Autodesk Inventor part; units mm, degrees
(part 2 of 5)
  spline S151 degree 2 poles (-398.6924, 73.057) (-398.9442, 73.057) (-399.3064, 73.4191) (-399.3064, 73.6794) knots 0 0 0 1 2 2 2
  spline S152 degree 2 poles (-399.3064, 73.6794) (-399.3064, 73.9312) (-398.9499, 74.2934) (-398.6924, 74.2934) knots 0 0 0 1 2 2 2
  spline S153 degree 2 poles (-398.6924, 74.2934) (-398.4293, 74.2934) (-398.07, 73.9256) (-398.07, 73.6794) knots 0 0 0 1 2 2 2
  line L183 (-388.2805, 72.641) -> (-388.4135, 73.2013)
  line L184 (-388.4135, 73.2013) -> (-389.3246, 73.2013)
  line L185 (-389.3246, 73.2013) -> (-389.4689, 72.641)
  line L186 (-389.4689, 72.641) -> (-390.4619, 72.641)
  line L187 (-390.4619, 72.641) -> (-389.4123, 75.691)
  line L188 (-389.4123, 75.691) -> (-388.2721, 75.691)
  line L189 (-388.2721, 75.691) -> (-387.2818, 72.641)
  line L190 (-387.2818, 72.641) -> (-388.2805, 72.641)
  line L191 (-388.8577, 75.0262) -> (-388.8775, 75.0262)
  spline S154 degree 2 poles (-388.8775, 75.0262) (-388.8832, 74.9752) (-388.9341, 74.7404) (-389.1661, 73.8548) knots 0 0 0 1 2 2 2
  line L192 (-389.1661, 73.8548) -> (-388.5833, 73.8548)
  line L193 (-388.5833, 73.8548) -> (-388.7955, 74.6838)
  spline S155 degree 2 poles (-388.7955, 74.6838) (-388.8407, 74.8677) (-388.8577, 75.0262) knots 0 0 0 1 1 1
  line L194 (-385.5955, 72.641) -> (-385.5955, 73.8294)
  spline S156 degree 2 poles (-385.5955, 73.8294) (-385.5955, 74.0331) (-385.7172, 74.2085) (-385.853, 74.2085) knots 0 0 0 1 2 2 2
  spline S157 degree 2 poles (-385.853, 74.2085) (-385.969, 74.2085) (-386.102, 74.0246) (-386.102, 73.8831) knots 0 0 0 1 2 2 2
  line L195 (-386.102, 73.8831) -> (-386.102, 72.641)
  line L196 (-386.102, 72.641) -> (-387.0074, 72.641)
  line L197 (-387.0074, 72.641) -> (-387.0074, 74.8196)
  line L198 (-387.0074, 74.8196) -> (-386.102, 74.8196)
  line L199 (-386.102, 74.8196) -> (-386.102, 74.4801)
  line L200 (-386.102, 74.4801) -> (-386.0935, 74.4801)
  spline S158 degree 2 poles (-386.0935, 74.4801) (-385.986, 74.6668) (-385.6182, 74.8734) (-385.4031, 74.8734) knots 0 0 0 1 2 2 2
  spline S159 degree 2 poles (-385.4031, 74.8734) (-384.6901, 74.8734) (-384.6901, 73.9708) knots 0 0 0 1 1 1
  line L201 (-384.6901, 73.9708) -> (-384.6901, 72.641)
  line L202 (-384.6901, 72.641) -> (-385.5955, 72.641)
  spline S160 degree 2 poles (-381.9174, 72.9438) (-381.9174, 72.3157) (-382.7068, 71.6168) (-383.465, 71.6168) knots 0 0 0 1 2 2 2
  spline S161 degree 2 poles (-383.465, 71.6168) (-383.6688, 71.6168) (-384.0535, 71.6819) (-384.1356, 71.7215) knots 0 0 0 1 2 2 2
  line L203 (-384.1356, 71.7215) -> (-384.1356, 72.4317)
  spline S162 degree 2 poles (-384.1356, 72.4317) (-383.9998, 72.3468) (-383.632, 72.2449) (-383.4905, 72.2449) knots 0 0 0 1 2 2 2
  spline S163 degree 2 poles (-383.4905, 72.2449) (-383.1849, 72.2449) (-382.82, 72.5392) (-382.82, 72.7825) knots 0 0 0 1 2 2 2
  line L204 (-382.82, 72.7825) -> (-382.82, 72.9155)
  line L205 (-382.82, 72.9155) -> (-382.8285, 72.9155)
  spline S164 degree 2 poles (-382.8285, 72.9155) (-382.9275, 72.7655) (-383.2698, 72.5873) (-383.465, 72.5873) knots 0 0 0 1 2 2 2
  spline S165 degree 2 poles (-383.465, 72.5873) (-383.8866, 72.5873) (-384.3761, 73.173) (-384.3761, 73.6879) knots 0 0 0 1 2 2 2
  spline S166 degree 2 poles (-384.3761, 73.6879) (-384.3761, 74.0416) (-384.1215, 74.582) (-383.6659, 74.8734) (-383.3915, 74.8734) knots 0 0 0 1 2 3 3 3
  spline S167 degree 2 poles (-383.3915, 74.8734) (-383.0124, 74.8734) (-382.8285, 74.5933) knots 0 0 0 1 1 1
  line L206 (-382.8285, 74.5933) -> (-382.82, 74.5933)
  line L207 (-382.82, 74.5933) -> (-382.82, 74.8196)
  line L208 (-382.82, 74.8196) -> (-381.9174, 74.8196)
  line L209 (-381.9174, 74.8196) -> (-381.9174, 72.9438)
  spline S168 degree 2 poles (-382.8058, 73.7926) (-382.8058, 73.9821) (-382.9784, 74.2085) (-383.1199, 74.2085) knots 0 0 0 1 2 2 2
  spline S169 degree 2 poles (-383.1199, 74.2085) (-383.2727, 74.2085) (-383.4566, 73.9369) (-383.4566, 73.7077) knots 0 0 0 1 2 2 2
  spline S170 degree 2 poles (-383.4566, 73.7077) (-383.4566, 73.4983) (-383.3038, 73.2522) (-383.1368, 73.2522) knots 0 0 0 1 2 2 2
  spline S171 degree 2 poles (-383.1368, 73.2522) (-382.9812, 73.2522) (-382.8058, 73.504) (-382.8058, 73.719) knots 0 0 0 1 2 2 2
  line L210 (-382.8058, 73.719) -> (-382.8058, 73.7926)
  spline S172 degree 2 poles (-380.7008, 73.4729) (-380.6782, 73.3314) (-380.4009, 73.173) (-380.1746, 73.173) knots 0 0 0 1 2 2 2
  spline S173 degree 2 poles (-380.1746, 73.173) (-379.8577, 73.173) (-379.5747, 73.2946) knots 0 0 0 1 1 1
  line L211 (-379.5747, 73.2946) -> (-379.5747, 72.7203)
  spline S174 degree 2 poles (-379.5747, 72.7203) (-379.9029, 72.5873) (-380.3754, 72.5873) knots 0 0 0 1 1 1
  spline S175 degree 2 poles (-380.3754, 72.5873) (-380.9441, 72.5873) (-381.5779, 73.1701) (-381.5779, 73.6822) knots 0 0 0 1 2 2 2
  spline S176 degree 2 poles (-381.5779, 73.6822) (-381.5779, 74.0331) (-381.3006, 74.5678) (-380.7546, 74.8734) (-380.4235, 74.8734) knots 0 0 0 1 2 3 3 3
  spline S177 degree 2 poles (-380.4235, 74.8734) (-380.0868, 74.8734) (-379.6059, 74.6103) (-379.3569, 74.1321) (-379.3569, 73.8124) knots 0 0 0 1 2 3 3 3
  line L212 (-379.3569, 73.8124) -> (-379.3569, 73.4729)
  line L213 (-379.3569, 73.4729) -> (-380.7008, 73.4729)
  spline S178 degree 2 poles (-380.1576, 73.9482) (-380.1576, 74.3245) (-380.4264, 74.3245) knots 0 0 0 1 1 1
  spline S179 degree 2 poles (-380.4264, 74.3245) (-380.5395, 74.3245) (-380.6923, 74.118) (-380.7065, 73.9482) knots 0 0 0 1 2 2 2
  line L214 (-380.7065, 73.9482) -> (-380.1576, 73.9482)
  line L215 (-379.0428, 72.641) -> (-379.0428, 75.8665)
  line L216 (-379.0428, 75.8665) -> (-378.1375, 75.8665)
  line L217 (-378.1375, 75.8665) -> (-378.1375, 72.641)
  line L218 (-378.1375, 72.641) -> (-379.0428, 72.641)
  spline S180 degree 2 poles (-375.2798, 73.7699) (-375.2798, 73.2182) (-375.9447, 72.5873) (-376.5417, 72.5873) knots 0 0 0 1 2 2 2
  spline S181 degree 2 poles (-376.5417, 72.5873) (-377.1359, 72.5873) (-377.7979, 73.2013) (-377.7979, 73.7445) knots 0 0 0 1 2 2 2
  spline S182 degree 2 poles (-377.7979, 73.7445) (-377.7979, 74.0897) (-377.4867, 74.6018) (-376.9124, 74.8734) (-376.5389, 74.8734) knots 0 0 0 1 2 3 3 3
  spline S183 degree 2 poles (-376.5389, 74.8734) (-376.1513, 74.8734) (-375.5826, 74.5876) (-375.2798, 74.0812) (-375.2798, 73.7699) knots 0 0 0 1 2 3 3 3
  spline S184 degree 2 poles (-376.1994, 73.7643) (-376.1994, 74.2085) (-376.5389, 74.2085) knots 0 0 0 1 1 1
  spline S185 degree 2 poles (-376.5389, 74.2085) (-376.8784, 74.2085) (-376.8784, 73.7445) knots 0 0 0 1 1 1
  spline S186 degree 2 poles (-376.8784, 73.7445) (-376.8784, 73.2522) (-376.5332, 73.2522) knots 0 0 0 1 1 1
  spline S187 degree 2 poles (-376.5332, 73.2522) (-376.1994, 73.2522) (-376.1994, 73.7643) knots 0 0 0 1 1 1
  line L219 (-373.5285, 72.641) -> (-373.5285, 73.8294)
  spline S188 degree 2 poles (-373.5285, 73.8294) (-373.5285, 74.0331) (-373.6502, 74.2085) (-373.786, 74.2085) knots 0 0 0 1 2 2 2
  spline S189 degree 2 poles (-373.786, 74.2085) (-373.902, 74.2085) (-374.0349, 74.0246) (-374.0349, 73.8831) knots 0 0 0 1 2 2 2
  line L220 (-374.0349, 73.8831) -> (-374.0349, 72.641)
  line L221 (-374.0349, 72.641) -> (-374.9403, 72.641)
  line L222 (-374.9403, 72.641) -> (-374.9403, 74.8196)
  line L223 (-374.9403, 74.8196) -> (-374.0349, 74.8196)
  line L224 (-374.0349, 74.8196) -> (-374.0349, 74.4801)
  line L225 (-374.0349, 74.4801) -> (-374.0265, 74.4801)
  spline S190 degree 2 poles (-374.0265, 74.4801) (-373.9189, 74.6668) (-373.5511, 74.8734) (-373.3361, 74.8734) knots 0 0 0 1 2 2 2
  spline S191 degree 2 poles (-373.3361, 74.8734) (-372.6231, 74.8734) (-372.6231, 73.9708) knots 0 0 0 1 1 1
  line L226 (-372.6231, 73.9708) -> (-372.6231, 72.641)
  line L227 (-372.6231, 72.641) -> (-373.5285, 72.641)
  line L228 (-372.2129, 72.641) -> (-372.2129, 74.8196)
  line L229 (-372.2129, 74.8196) -> (-371.3075, 74.8196)
  line L230 (-371.3075, 74.8196) -> (-371.3075, 72.641)
  line L231 (-371.3075, 72.641) -> (-372.2129, 72.641)
  spline S192 degree 2 poles (-371.2537, 75.4081) (-371.2537, 75.2157) (-371.5338, 74.9781) (-371.7602, 74.9781) knots 0 0 0 1 2 2 2
  spline S193 degree 2 poles (-371.7602, 74.9781) (-371.9809, 74.9781) (-372.2638, 75.2242) (-372.2638, 75.4081) knots 0 0 0 1 2 2 2
  spline S194 degree 2 poles (-372.2638, 75.4081) (-372.2638, 75.5949) (-371.9894, 75.8269) (-371.7602, 75.8269) knots 0 0 0 1 2 2 2
  spline S195 degree 2 poles (-371.7602, 75.8269) (-371.5338, 75.8269) (-371.2537, 75.5949) (-371.2537, 75.4081) knots 0 0 0 1 2 2 2
  line L232 (-369.5788, 72.641) -> (-369.5788, 75.691)
  line L233 (-369.5788, 75.691) -> (-368.6593, 75.691)
  line L234 (-368.6593, 75.691) -> (-368.6593, 72.641)
  line L235 (-368.6593, 72.641) -> (-369.5788, 72.641)
  line L236 (-368.1415, 72.641) -> (-368.1415, 75.8665)
  line L237 (-368.1415, 75.8665) -> (-367.2361, 75.8665)
  line L238 (-367.2361, 75.8665) -> (-367.2361, 72.641)
  line L239 (-367.2361, 72.641) -> (-368.1415, 72.641)
  line L240 (-365.5923, 72.641) -> (-365.5923, 72.9721)
  line L241 (-365.5923, 72.9721) -> (-365.6008, 72.9721)
  spline S196 degree 2 poles (-365.6008, 72.9721) (-365.8186, 72.5873) (-366.2657, 72.5873) knots 0 0 0 1 1 1
  spline S197 degree 2 poles (-366.2657, 72.5873) (-366.574, 72.5873) (-366.9221, 72.9523) (-366.9221, 73.2607) knots 0 0 0 1 2 2 2
  spline S198 degree 2 poles (-366.9221, 73.2607) (-366.9221, 73.9029) (-366.1327, 74.0048) knots 0 0 0 1 1 1
  line L242 (-366.1327, 74.0048) -> (-365.5923, 74.0755)
  spline S199 degree 2 poles (-365.5923, 74.0755) (-365.5923, 74.183) (-365.7847, 74.3188) (-365.9459, 74.3188) knots 0 0 0 1 2 2 2
  spline S200 degree 2 poles (-365.9459, 74.3188) (-366.3109, 74.3188) (-366.7183, 74.1095) knots 0 0 0 1 1 1
  line L243 (-366.7183, 74.1095) -> (-366.7183, 74.698)
  spline S201 degree 2 poles (-366.7183, 74.698) (-366.5429, 74.7744) (-366.0082, 74.8734) (-365.8186, 74.8734) knots 0 0 0 1 2 2 2
  spline S202 degree 2 poles (-365.8186, 74.8734) (-365.2641, 74.8734) (-364.7633, 74.3981) (-364.7633, 73.8435) knots 0 0 0 1 2 2 2
  line L244 (-364.7633, 73.8435) -> (-364.7633, 72.641)
  line L245 (-364.7633, 72.641) -> (-365.5923, 72.641)
  spline S203 degree 2 poles (-366.1298, 73.3823) (-366.1298, 73.2946) (-366.0167, 73.1786) (-365.912, 73.1786) knots 0 0 0 1 2 2 2
  spline S204 degree 2 poles (-365.912, 73.1786) (-365.7705, 73.1786) (-365.5923, 73.3908) (-365.5923, 73.5577) knots 0 0 0 1 2 2 2
  line L246 (-365.5923, 73.5577) -> (-365.5923, 73.6398)
  line L247 (-365.5923, 73.6398) -> (-365.9007, 73.5974)
  spline S205 degree 2 poles (-365.9007, 73.5974) (-366.1298, 73.5577) (-366.1298, 73.3823) knots 0 0 0 1 1 1
  spline S206 degree 2 poles (-362.7177, 74.0444) (-362.7686, 74.067) (-362.944, 74.1038) (-363.0006, 74.1038) knots 0 0 0 1 2 2 2
  spline S207 degree 2 poles (-363.0006, 74.1038) (-363.4505, 74.1038) (-363.4505, 73.586) knots 0 0 0 1 1 1
  line L248 (-363.4505, 73.586) -> (-363.4505, 72.641)
  line L249 (-363.4505, 72.641) -> (-364.3559, 72.641)
  line L250 (-364.3559, 72.641) -> (-364.3559, 74.8196)
  line L251 (-364.3559, 74.8196) -> (-363.4505, 74.8196)
  line L252 (-363.4505, 74.8196) -> (-363.4505, 74.4377)
  line L253 (-363.4505, 74.4377) -> (-363.442, 74.4377)
  spline S208 degree 2 poles (-363.442, 74.4377) (-363.3599, 74.6442) (-363.0516, 74.8592) (-362.8478, 74.8592) knots 0 0 0 1 2 2 2
  spline S209 degree 2 poles (-362.8478, 74.8592) (-362.7743, 74.8592) (-362.7177, 74.8338) knots 0 0 0 1 1 1
  line L254 (-362.7177, 74.8338) -> (-362.7177, 74.0444)
  line L255 (-362.4574, 72.641) -> (-362.4574, 74.8196)
  line L256 (-362.4574, 74.8196) -> (-361.552, 74.8196)
  line L257 (-361.552, 74.8196) -> (-361.552, 72.641)
  line L258 (-361.552, 72.641) -> (-362.4574, 72.641)
  spline S210 degree 2 poles (-361.4983, 75.4081) (-361.4983, 75.2157) (-361.7784, 74.9781) (-362.0047, 74.9781) knots 0 0 0 1 2 2 2
  spline S211 degree 2 poles (-362.0047, 74.9781) (-362.2254, 74.9781) (-362.5083, 75.2242) (-362.5083, 75.4081) knots 0 0 0 1 2 2 2
  spline S212 degree 2 poles (-362.5083, 75.4081) (-362.5083, 75.5949) (-362.2339, 75.8269) (-362.0047, 75.8269) knots 0 0 0 1 2 2 2
  spline S213 degree 2 poles (-362.0047, 75.8269) (-361.7784, 75.8269) (-361.4983, 75.5949) (-361.4983, 75.4081) knots 0 0 0 1 2 2 2
  line L259 (-359.9082, 72.641) -> (-359.9082, 72.9721)
  line L260 (-359.9082, 72.9721) -> (-359.9167, 72.9721)
  spline S214 degree 2 poles (-359.9167, 72.9721) (-360.1345, 72.5873) (-360.5816, 72.5873) knots 0 0 0 1 1 1
  spline S215 degree 2 poles (-360.5816, 72.5873) (-360.89, 72.5873) (-361.238, 72.9523) (-361.238, 73.2607) knots 0 0 0 1 2 2 2
  spline S216 degree 2 poles (-361.238, 73.2607) (-361.238, 73.9029) (-360.4486, 74.0048) knots 0 0 0 1 1 1
  line L261 (-360.4486, 74.0048) -> (-359.9082, 74.0755)
  spline S217 degree 2 poles (-359.9082, 74.0755) (-359.9082, 74.183) (-360.1006, 74.3188) (-360.2618, 74.3188) knots 0 0 0 1 2 2 2
  spline S218 degree 2 poles (-360.2618, 74.3188) (-360.6268, 74.3188) (-361.0343, 74.1095) knots 0 0 0 1 1 1
  line L262 (-361.0343, 74.1095) -> (-361.0343, 74.698)
  spline S219 degree 2 poles (-361.0343, 74.698) (-360.8588, 74.7744) (-360.3241, 74.8734) (-360.1345, 74.8734) knots 0 0 0 1 2 2 2
  spline S220 degree 2 poles (-360.1345, 74.8734) (-359.58, 74.8734) (-359.0792, 74.3981) (-359.0792, 73.8435) knots 0 0 0 1 2 2 2
  line L263 (-359.0792, 73.8435) -> (-359.0792, 72.641)
  line L264 (-359.0792, 72.641) -> (-359.9082, 72.641)
  spline S221 degree 2 poles (-360.4458, 73.3823) (-360.4458, 73.2946) (-360.3326, 73.1786) (-360.2279, 73.1786) knots 0 0 0 1 2 2 2
  spline S222 degree 2 poles (-360.2279, 73.1786) (-360.0864, 73.1786) (-359.9082, 73.3908) (-359.9082, 73.5577) knots 0 0 0 1 2 2 2
  line L265 (-359.9082, 73.5577) -> (-359.9082, 73.6398)
  line L266 (-359.9082, 73.6398) -> (-360.2166, 73.5974)
  spline S223 degree 2 poles (-360.2166, 73.5974) (-360.4458, 73.5577) (-360.4458, 73.3823) knots 0 0 0 1 1 1
  spline S224 degree 2 poles (-398.07, 67.7427) (-398.07, 67.5786) (-398.2397, 67.2872) (-398.5311, 67.1203) (-398.6924, 67.1203) knots 0 0 0 1 2 3 3 3
  spline S225 degree 2 poles (-398.6924, 67.1203) (-398.9442, 67.1203) (-399.3064, 67.4824) (-399.3064, 67.7427) knots 0 0 0 1 2 2 2
  spline S226 degree 2 poles (-399.3064, 67.7427) (-399.3064, 67.9946) (-398.9499, 68.3567) (-398.6924, 68.3567) knots 0 0 0 1 2 2 2
  spline S227 degree 2 poles (-398.6924, 68.3567) (-398.4293, 68.3567) (-398.07, 67.9889) (-398.07, 67.7427) knots 0 0 0 1 2 2 2
  line L267 (-388.2805, 66.7044) -> (-388.4135, 67.2646)
  line L268 (-388.4135, 67.2646) -> (-389.3246, 67.2646)
  line L269 (-389.3246, 67.2646) -> (-389.4689, 66.7044)
  line L270 (-389.4689, 66.7044) -> (-390.4619, 66.7044)
  line L271 (-390.4619, 66.7044) -> (-389.4123, 69.7544)
  line L272 (-389.4123, 69.7544) -> (-388.2721, 69.7544)
  line L273 (-388.2721, 69.7544) -> (-387.2818, 66.7044)
  line L274 (-387.2818, 66.7044) -> (-388.2805, 66.7044)
  line L275 (-388.8577, 69.0895) -> (-388.8775, 69.0895)
  spline S228 degree 2 poles (-388.8775, 69.0895) (-388.8832, 69.0386) (-388.9341, 68.8037) (-389.1661, 67.9182) knots 0 0 0 1 2 2 2
  line L276 (-389.1661, 67.9182) -> (-388.5833, 67.9182)
  line L277 (-388.5833, 67.9182) -> (-388.7955, 68.7471)
  spline S229 degree 2 poles (-388.7955, 68.7471) (-388.8407, 68.9311) (-388.8577, 69.0895) knots 0 0 0 1 1 1
  line L278 (-385.5955, 66.7044) -> (-385.5955, 67.8927)
  spline S230 degree 2 poles (-385.5955, 67.8927) (-385.5955, 68.0964) (-385.7172, 68.2718) (-385.853, 68.2718) knots 0 0 0 1 2 2 2
  spline S231 degree 2 poles (-385.853, 68.2718) (-385.969, 68.2718) (-386.102, 68.0879) (-386.102, 67.9465) knots 0 0 0 1 2 2 2
  line L279 (-386.102, 67.9465) -> (-386.102, 66.7044)
  line L280 (-386.102, 66.7044) -> (-387.0074, 66.7044)
  line L281 (-387.0074, 66.7044) -> (-387.0074, 68.883)
  line L282 (-387.0074, 68.883) -> (-386.102, 68.883)
  line L283 (-386.102, 68.883) -> (-386.102, 68.5434)
  line L284 (-386.102, 68.5434) -> (-386.0935, 68.5434)
  spline S232 degree 2 poles (-386.0935, 68.5434) (-385.986, 68.7302) (-385.6182, 68.9367) (-385.4031, 68.9367) knots 0 0 0 1 2 2 2
  spline S233 degree 2 poles (-385.4031, 68.9367) (-384.6901, 68.9367) (-384.6901, 68.0342) knots 0 0 0 1 1 1
  line L285 (-384.6901, 68.0342) -> (-384.6901, 66.7044)
  line L286 (-384.6901, 66.7044) -> (-385.5955, 66.7044)
  spline S234 degree 2 poles (-382.7464, 66.7327) (-382.8086, 66.7044) (-383.0888, 66.6506) (-383.2868, 66.6506) knots 0 0 0 1 2 2 2
  spline S235 degree 2 poles (-383.2868, 66.6506) (-383.6659, 66.6506) (-384.0932, 67.0665) (-384.0932, 67.4542) knots 0 0 0 1 2 2 2
  line L287 (-384.0932, 67.4542) -> (-384.0932, 68.2548)
  line L288 (-384.0932, 68.2548) -> (-384.4355, 68.2548)
  line L289 (-384.4355, 68.2548) -> (-384.4355, 68.883)
  line L290 (-384.4355, 68.883) -> (-384.0932, 68.883)
  line L291 (-384.0932, 68.883) -> (-384.0932, 69.3102)
  line L292 (-384.0932, 69.3102) -> (-383.1991, 69.5563)
  line L293 (-383.1991, 69.5563) -> (-383.1991, 68.883)
  line L294 (-383.1991, 68.883) -> (-382.7464, 68.883)
  line L295 (-382.7464, 68.883) -> (-382.7464, 68.2548)
  line L296 (-382.7464, 68.2548) -> (-383.1991, 68.2548)
  line L297 (-383.1991, 68.2548) -> (-383.1991, 67.6013)
  spline S236 degree 2 poles (-383.1991, 67.6013) (-383.1991, 67.3155) (-382.9727, 67.3155) knots 0 0 0 1 1 1
  spline S237 degree 2 poles (-382.9727, 67.3155) (-382.8652, 67.3155) (-382.7464, 67.3608) knots 0 0 0 1 1 1
  line L298 (-382.7464, 67.3608) -> (-382.7464, 66.7327)
  spline S238 degree 2 poles (-380.0416, 67.8333) (-380.0416, 67.2816) (-380.7065, 66.6506) (-381.3035, 66.6506) knots 0 0 0 1 2 2 2
  spline S239 degree 2 poles (-381.3035, 66.6506) (-381.8976, 66.6506) (-382.5597, 67.2646) (-382.5597, 67.8078) knots 0 0 0 1 2 2 2
  spline S240 degree 2 poles (-382.5597, 67.8078) (-382.5597, 68.153) (-382.2484, 68.6651) (-381.6741, 68.9367) (-381.3006, 68.9367) knots 0 0 0 1 2 3 3 3
  spline S241 degree 2 poles (-381.3006, 68.9367) (-380.913, 68.9367) (-380.3443, 68.651) (-380.0416, 68.1445) (-380.0416, 67.8333) knots 0 0 0 1 2 3 3 3
  spline S242 degree 2 poles (-380.9611, 67.8276) (-380.9611, 68.2718) (-381.3006, 68.2718) knots 0 0 0 1 1 1
  spline S243 degree 2 poles (-381.3006, 68.2718) (-381.6401, 68.2718) (-381.6401, 67.8078) knots 0 0 0 1 1 1
  spline S244 degree 2 poles (-381.6401, 67.8078) (-381.6401, 67.3155) (-381.295, 67.3155) knots 0 0 0 1 1 1
  spline S245 degree 2 poles (-381.295, 67.3155) (-380.9611, 67.3155) (-380.9611, 67.8276) knots 0 0 0 1 1 1
  line L299 (-378.2902, 66.7044) -> (-378.2902, 67.8927)
  spline S246 degree 2 poles (-378.2902, 67.8927) (-378.2902, 68.0964) (-378.4119, 68.2718) (-378.5477, 68.2718) knots 0 0 0 1 2 2 2
  spline S247 degree 2 poles (-378.5477, 68.2718) (-378.6637, 68.2718) (-378.7967, 68.0879) (-378.7967, 67.9465) knots 0 0 0 1 2 2 2
  line L300 (-378.7967, 67.9465) -> (-378.7967, 66.7044)
  line L301 (-378.7967, 66.7044) -> (-379.7021, 66.7044)
  line L302 (-379.7021, 66.7044) -> (-379.7021, 68.883)
  line L303 (-379.7021, 68.883) -> (-378.7967, 68.883)
  line L304 (-378.7967, 68.883) -> (-378.7967, 68.5434)
  line L305 (-378.7967, 68.5434) -> (-378.7882, 68.5434)
  spline S248 degree 2 poles (-378.7882, 68.5434) (-378.6807, 68.7302) (-378.3129, 68.9367) (-378.0978, 68.9367) knots 0 0 0 1 2 2 2
  spline S249 degree 2 poles (-378.0978, 68.9367) (-377.3849, 68.9367) (-377.3849, 68.0342) knots 0 0 0 1 1 1
  line L306 (-377.3849, 68.0342) -> (-377.3849, 66.7044)
  line L307 (-377.3849, 66.7044) -> (-378.2902, 66.7044)
  line L308 (-376.9746, 66.7044) -> (-376.9746, 68.883)
  line L309 (-376.9746, 68.883) -> (-376.0692, 68.883)
  line L310 (-376.0692, 68.883) -> (-376.0692, 66.7044)
  line L311 (-376.0692, 66.7044) -> (-376.9746, 66.7044)
  spline S250 degree 2 poles (-376.0155, 69.4715) (-376.0155, 69.2791) (-376.2956, 69.0414) (-376.5219, 69.0414) knots 0 0 0 1 2 2 2
  spline S251 degree 2 poles (-376.5219, 69.0414) (-376.7426, 69.0414) (-377.0255, 69.2875) (-377.0255, 69.4715) knots 0 0 0 1 2 2 2
  spline S252 degree 2 poles (-377.0255, 69.4715) (-377.0255, 69.6582) (-376.7511, 69.8902) (-376.5219, 69.8902) knots 0 0 0 1 2 2 2
  spline S253 degree 2 poles (-376.5219, 69.8902) (-376.2956, 69.8902) (-376.0155, 69.6582) (-376.0155, 69.4715) knots 0 0 0 1 2 2 2
  line L312 (-374.2217, 66.7044) -> (-374.2217, 67.8927)
  spline S254 degree 2 poles (-374.2217, 67.8927) (-374.2217, 68.0964) (-374.3433, 68.2718) (-374.4791, 68.2718) knots 0 0 0 1 2 2 2
  spline S255 degree 2 poles (-374.4791, 68.2718) (-374.5952, 68.2718) (-374.7281, 68.0879) (-374.7281, 67.9465) knots 0 0 0 1 2 2 2
  line L313 (-374.7281, 67.9465) -> (-374.7281, 66.7044)
  line L314 (-374.7281, 66.7044) -> (-375.6335, 66.7044)
  line L315 (-375.6335, 66.7044) -> (-375.6335, 68.883)
  line L316 (-375.6335, 68.883) -> (-374.7281, 68.883)
  line L317 (-374.7281, 68.883) -> (-374.7281, 68.5434)
  line L318 (-374.7281, 68.5434) -> (-374.7196, 68.5434)
  spline S256 degree 2 poles (-374.7196, 68.5434) (-374.6121, 68.7302) (-374.2443, 68.9367) (-374.0293, 68.9367) knots 0 0 0 1 2 2 2
  spline S257 degree 2 poles (-374.0293, 68.9367) (-373.3163, 68.9367) (-373.3163, 68.0342) knots 0 0 0 1 1 1
  line L319 (-373.3163, 68.0342) -> (-373.3163, 66.7044)
  line L320 (-373.3163, 66.7044) -> (-374.2217, 66.7044)
  line L321 (-372.9061, 66.7044) -> (-372.9061, 68.883)
  line L322 (-372.9061, 68.883) -> (-372.0007, 68.883)
  line L323 (-372.0007, 68.883) -> (-372.0007, 66.7044)
  line L324 (-372.0007, 66.7044) -> (-372.9061, 66.7044)
  spline S258 degree 2 poles (-371.9469, 69.4715) (-371.9469, 69.2791) (-372.227, 69.0414) (-372.4534, 69.0414) knots 0 0 0 1 2 2 2
  spline S259 degree 2 poles (-372.4534, 69.0414) (-372.674, 69.0414) (-372.957, 69.2875) (-372.957, 69.4715) knots 0 0 0 1 2 2 2
  spline S260 degree 2 poles (-372.957, 69.4715) (-372.957, 69.6582) (-372.6825, 69.8902) (-372.4534, 69.8902) knots 0 0 0 1 2 2 2
  spline S261 degree 2 poles (-372.4534, 69.8902) (-372.227, 69.8902) (-371.9469, 69.6582) (-371.9469, 69.4715) knots 0 0 0 1 2 2 2
  spline S262 degree 2 poles (-367.3945, 68.269) (-367.3945, 67.805) (-367.785, 67.092) (-368.5065, 66.7044) (-368.979, 66.7044) knots 0 0 0 1 2 3 3 3
  line L325 (-368.979, 66.7044) -> (-370.272, 66.7044)
  line L326 (-370.272, 66.7044) -> (-370.272, 69.7544)
  line L327 (-370.272, 69.7544) -> (-369.0073, 69.7544)
  spline S263 degree 2 poles (-369.0073, 69.7544) (-367.3945, 69.7544) (-367.3945, 68.269) knots 0 0 0 1 1 1
  spline S264 degree 2 poles (-368.3707, 68.2605) (-368.3707, 68.4812) (-368.5517, 68.8405) (-368.8884, 69.0357) (-369.1148, 69.0357) knots 0 0 0 1 2 3 3 3
  line L328 (-369.1148, 69.0357) -> (-369.3524, 69.0357)
  line L329 (-369.3524, 69.0357) -> (-369.3524, 67.423)
  line L330 (-369.3524, 67.423) -> (-369.095, 67.423)
  spline S265 degree 2 poles (-369.095, 67.423) (-368.7639, 67.423) (-368.3707, 67.8757) (-368.3707, 68.2605) knots 0 0 0 1 2 2 2
  line L331 (-365.8384, 66.7044) -> (-365.8384, 67.0354)
  line L332 (-365.8384, 67.0354) -> (-365.8469, 67.0354)
  spline S266 degree 2 poles (-365.8469, 67.0354) (-366.0648, 66.6506) (-366.5118, 66.6506) knots 0 0 0 1 1 1
  spline S267 degree 2 poles (-366.5118, 66.6506) (-366.8202, 66.6506) (-367.1682, 67.0156) (-367.1682, 67.324) knots 0 0 0 1 2 2 2
  spline S268 degree 2 poles (-367.1682, 67.324) (-367.1682, 67.9663) (-366.3788, 68.0681) knots 0 0 0 1 1 1
  line L333 (-366.3788, 68.0681) -> (-365.8384, 68.1388)
  spline S269 degree 2 poles (-365.8384, 68.1388) (-365.8384, 68.2464) (-366.0308, 68.3822) (-366.1921, 68.3822) knots 0 0 0 1 2 2 2
  spline S270 degree 2 poles (-366.1921, 68.3822) (-366.5571, 68.3822) (-366.9645, 68.1728) knots 0 0 0 1 1 1
  line L334 (-366.9645, 68.1728) -> (-366.9645, 68.7613)
  spline S271 degree 2 poles (-366.9645, 68.7613) (-366.7891, 68.8377) (-366.2543, 68.9367) (-366.0648, 68.9367) knots 0 0 0 1 2 2 2
  spline S272 degree 2 poles (-366.0648, 68.9367) (-365.5102, 68.9367) (-365.0094, 68.4614) (-365.0094, 67.9068) knots 0 0 0 1 2 2 2
  line L335 (-365.0094, 67.9068) -> (-365.0094, 66.7044)
  line L336 (-365.0094, 66.7044) -> (-365.8384, 66.7044)
  spline S273 degree 2 poles (-366.376, 67.4457) (-366.376, 67.358) (-366.2628, 67.242) (-366.1581, 67.242) knots 0 0 0 1 2 2 2
  spline S274 degree 2 poles (-366.1581, 67.242) (-366.0167, 67.242) (-365.8384, 67.4542) (-365.8384, 67.6211) knots 0 0 0 1 2 2 2
  line L337 (-365.8384, 67.6211) -> (-365.8384, 67.7031)
  line L338 (-365.8384, 67.7031) -> (-366.1468, 67.6607)
  spline S275 degree 2 poles (-366.1468, 67.6607) (-366.376, 67.6211) (-366.376, 67.4457) knots 0 0 0 1 1 1
  line L339 (-363.0176, 66.7044) -> (-364.0927, 66.7044)
  line L340 (-364.0927, 66.7044) -> (-364.8199, 68.883)
  line L341 (-364.8199, 68.883) -> (-363.8749, 68.883)
  line L342 (-363.8749, 68.883) -> (-363.6089, 67.6946)
  spline S276 degree 2 poles (-363.6089, 67.6946) (-363.5467, 67.4061) (-363.5382, 67.2618) knots 0 0 0 1 1 1
  line L343 (-363.5382, 67.2618) -> (-363.5269, 67.2618)
  spline S277 degree 2 poles (-363.5269, 67.2618) (-363.5212, 67.3042) (-363.5071, 67.3947) (-363.1987, 68.883) knots 0 0 0 1 2 2 2
  line L344 (-363.1987, 68.883) -> (-362.2593, 68.883)
  line L345 (-362.2593, 68.883) -> (-363.0176, 66.7044)
  line L346 (-362.0415, 66.7044) -> (-362.0415, 68.883)
  line L347 (-362.0415, 68.883) -> (-361.1361, 68.883)
  line L348 (-361.1361, 68.883) -> (-361.1361, 66.7044)
  line L349 (-361.1361, 66.7044) -> (-362.0415, 66.7044)
  spline S278 degree 2 poles (-361.0823, 69.4715) (-361.0823, 69.2791) (-361.3625, 69.0414) (-361.5888, 69.0414) knots 0 0 0 1 2 2 2
  spline S279 degree 2 poles (-361.5888, 69.0414) (-361.8095, 69.0414) (-362.0924, 69.2875) (-362.0924, 69.4715) knots 0 0 0 1 2 2 2
  spline S280 degree 2 poles (-362.0924, 69.4715) (-362.0924, 69.6582) (-361.818, 69.8902) (-361.5888, 69.8902) knots 0 0 0 1 2 2 2
  spline S281 degree 2 poles (-361.5888, 69.8902) (-361.3625, 69.8902) (-361.0823, 69.6582) (-361.0823, 69.4715) knots 0 0 0 1 2 2 2
  line L350 (-359.2461, 66.7044) -> (-359.2461, 66.959)
  line L351 (-359.2461, 66.959) -> (-359.2546, 66.959)
  spline S282 degree 2 poles (-359.2546, 66.959) (-359.3621, 66.8147) (-359.713, 66.6506) (-359.8827, 66.6506) knots 0 0 0 1 2 2 2
  spline S283 degree 2 poles (-359.8827, 66.6506) (-360.16, 66.6506) (-360.5872, 66.9251) (-360.7966, 67.4202) (-360.7966, 67.7541) knots 0 0 0 1 2 3 3 3
  spline S284 degree 2 poles (-360.7966, 67.7541) (-360.7966, 68.1021) (-360.5448, 68.6396) (-360.0893, 68.9367) (-359.8063, 68.9367) knots 0 0 0 1 2 3 3 3
  spline S285 degree 2 poles (-359.8063, 68.9367) (-359.6734, 68.9367) (-359.447, 68.8603) (-359.2772, 68.7302) (-359.2546, 68.6651) knots 0 0 0 1 2 3 3 3
  line L352 (-359.2546, 68.6651) -> (-359.2461, 68.6651)
  line L353 (-359.2461, 68.6651) -> (-359.2461, 69.9298)
  line L354 (-359.2461, 69.9298) -> (-358.3407, 69.9298)
  line L355 (-358.3407, 69.9298) -> (-358.3407, 66.7044)
  line L356 (-358.3407, 66.7044) -> (-359.2461, 66.7044)
  spline S286 degree 2 poles (-359.2263, 67.8587) (-359.2263, 68.054) (-359.3989, 68.2718) (-359.546, 68.2718) knots 0 0 0 1 2 2 2
  spline S287 degree 2 poles (-359.546, 68.2718) (-359.6932, 68.2718) (-359.8771, 68.003) (-359.8771, 67.7767) knots 0 0 0 1 2 2 2
  spline S288 degree 2 poles (-359.8771, 67.7767) (-359.8771, 67.3155) (-359.5573, 67.3155) knots 0 0 0 1 1 1
  spline S289 degree 2 poles (-359.5573, 67.3155) (-359.4074, 67.3155) (-359.2263, 67.5645) (-359.2263, 67.8022) knots 0 0 0 1 2 2 2
  line L357 (-359.2263, 67.8022) -> (-359.2263, 67.8587)
  spline S290 degree 2 poles (-357.1213, 67.5362) (-357.0987, 67.3947) (-356.8214, 67.2363) (-356.5951, 67.2363) knots 0 0 0 1 2 2 2
  spline S291 degree 2 poles (-356.5951, 67.2363) (-356.2782, 67.2363) (-355.9952, 67.358) knots 0 0 0 1 1 1
  line L358 (-355.9952, 67.358) -> (-355.9952, 66.7836)
  spline S292 degree 2 poles (-355.9952, 66.7836) (-356.3234, 66.6506) (-356.7959, 66.6506) knots 0 0 0 1 1 1
  spline S293 degree 2 poles (-356.7959, 66.6506) (-357.3646, 66.6506) (-357.9984, 67.2335) (-357.9984, 67.7456) knots 0 0 0 1 2 2 2
  spline S294 degree 2 poles (-357.9984, 67.7456) (-357.9984, 68.0964) (-357.7211, 68.6311) (-357.1751, 68.9367) (-356.844, 68.9367) knots 0 0 0 1 2 3 3 3
  spline S295 degree 2 poles (-356.844, 68.9367) (-356.5073, 68.9367) (-356.0264, 68.6736) (-355.7774, 68.1954) (-355.7774, 67.8757) knots 0 0 0 1 2 3 3 3
  line L359 (-355.7774, 67.8757) -> (-355.7774, 67.5362)
  line L360 (-355.7774, 67.5362) -> (-357.1213, 67.5362)
  spline S296 degree 2 poles (-356.5781, 68.0115) (-356.5781, 68.3878) (-356.8469, 68.3878) knots 0 0 0 1 1 1
  spline S297 degree 2 poles (-356.8469, 68.3878) (-356.96, 68.3878) (-357.1128, 68.1813) (-357.127, 68.0115) knots 0 0 0 1 2 2 2
  line L361 (-357.127, 68.0115) -> (-356.5781, 68.0115)
  spline S298 degree 2 poles (-398.07, 61.8061) (-398.07, 61.642) (-398.2397, 61.3506) (-398.5311, 61.1836) (-398.6924, 61.1836) knots 0 0 0 1 2 3 3 3
  spline S299 degree 2 poles (-398.6924, 61.1836) (-398.9442, 61.1836) (-399.3064, 61.5458) (-399.3064, 61.8061) knots 0 0 0 1 2 2 2
  spline S300 degree 2 poles (-399.3064, 61.8061) (-399.3064, 62.0579) (-398.9499, 62.42) (-398.6924, 62.42) knots 0 0 0 1 2 2 2
  spline S301 degree 2 poles (-398.6924, 62.42) (-398.4293, 62.42) (-398.07, 62.0522) (-398.07, 61.8061) knots 0 0 0 1 2 2 2
  spline S302 degree 2 poles (-387.924, 60.8498) (-388.3032, 60.714) (-388.7983, 60.714) knots 0 0 0 1 1 1
  spline S303 degree 2 poles (-388.7983, 60.714) (-389.2849, 60.714) (-389.9894, 61.0874) (-390.3629, 61.7721) (-390.3629, 62.222) knots 0 0 0 1 2 3 3 3
  spline S304 degree 2 poles (-390.3629, 62.222) (-390.3629, 62.7058) (-389.947, 63.4584) (-389.1859, 63.8686) (-388.6908, 63.8686) knots 0 0 0 1 2 3 3 3
  spline S305 degree 2 poles (-388.6908, 63.8686) (-388.2947, 63.8686) (-387.924, 63.7725) knots 0 0 0 1 1 1
  line L362 (-387.924, 63.7725) -> (-387.924, 62.9237)
  spline S306 degree 2 poles (-387.924, 62.9237) (-388.0514, 63) (-388.405, 63.0849) (-388.5833, 63.0849) knots 0 0 0 1 2 2 2
  spline S307 degree 2 poles (-388.5833, 63.0849) (-388.9596, 63.0849) (-389.3896, 62.6549) (-389.3896, 62.2871) knots 0 0 0 1 2 2 2
  spline S308 degree 2 poles (-389.3896, 62.2871) (-389.3896, 61.9221) (-388.9596, 61.4977) (-388.5974, 61.4977) knots 0 0 0 1 2 2 2
  spline S309 degree 2 poles (-388.5974, 61.4977) (-388.2636, 61.4977) (-387.924, 61.6703) knots 0 0 0 1 1 1
  line L363 (-387.924, 61.6703) -> (-387.924, 60.8498)
  spline S310 degree 2 poles (-385.1089, 61.8966) (-385.1089, 61.3449) (-385.7738, 60.714) (-386.3708, 60.714) knots 0 0 0 1 2 2 2
  spline S311 degree 2 poles (-386.3708, 60.714) (-386.9649, 60.714) (-387.627, 61.3279) (-387.627, 61.8712) knots 0 0 0 1 2 2 2
  spline S312 degree 2 poles (-387.627, 61.8712) (-387.627, 62.2163) (-387.3157, 62.7284) (-386.7414, 63) (-386.3679, 63) knots 0 0 0 1 2 3 3 3
  spline S313 degree 2 poles (-386.3679, 63) (-385.9803, 63) (-385.4116, 62.7143) (-385.1089, 62.2078) (-385.1089, 61.8966) knots 0 0 0 1 2 3 3 3
  spline S314 degree 2 poles (-386.0284, 61.891) (-386.0284, 62.3352) (-386.3679, 62.3352) knots 0 0 0 1 1 1
  spline S315 degree 2 poles (-386.3679, 62.3352) (-386.7074, 62.3352) (-386.7074, 61.8712) knots 0 0 0 1 1 1
  spline S316 degree 2 poles (-386.7074, 61.8712) (-386.7074, 61.3789) (-386.3623, 61.3789) knots 0 0 0 1 1 1
  spline S317 degree 2 poles (-386.3623, 61.3789) (-386.0284, 61.3789) (-386.0284, 61.891) knots 0 0 0 1 1 1
  spline S318 degree 2 poles (-382.9982, 61.492) (-382.9982, 61.1214) (-383.5641, 60.714) (-384.0677, 60.714) knots 0 0 0 1 2 2 2
  spline S319 degree 2 poles (-384.0677, 60.714) (-384.2148, 60.714) (-384.6477, 60.7734) (-384.7835, 60.8158) knots 0 0 0 1 2 2 2
  line L364 (-384.7835, 60.8158) -> (-384.7835, 61.4524)
  spline S320 degree 2 poles (-384.7835, 61.4524) (-384.3817, 61.2742) (-384.1101, 61.2742) knots 0 0 0 1 1 1
  spline S321 degree 2 poles (-384.1101, 61.2742) (-383.8442, 61.2742) (-383.8442, 61.4128) knots 0 0 0 1 1 1
  spline S322 degree 2 poles (-383.8442, 61.4128) (-383.8442, 61.4694) (-383.9687, 61.5458) (-384.229, 61.6307) knots 0 0 0 1 2 2 2
  spline S323 degree 2 poles (-384.229, 61.6307) (-384.5204, 61.724) (-384.7835, 62.0268) (-384.7835, 62.2673) knots 0 0 0 1 2 2 2
  spline S324 degree 2 poles (-384.7835, 62.2673) (-384.7835, 62.6068) (-384.2431, 63) (-383.7565, 63) knots 0 0 0 1 2 2 2
  spline S325 degree 2 poles (-383.7565, 63) (-383.4707, 63) (-383.151, 62.918) knots 0 0 0 1 1 1
  line L365 (-383.151, 62.918) -> (-383.151, 62.3069)
  spline S326 degree 2 poles (-383.151, 62.3069) (-383.2868, 62.3635) (-383.6065, 62.4398) (-383.714, 62.4398) knots 0 0 0 1 2 2 2
  spline S327 degree 2 poles (-383.714, 62.4398) (-383.8046, 62.4398) (-383.9121, 62.3804) (-383.9121, 62.3267) knots 0 0 0 1 2 2 2
  spline S328 degree 2 poles (-383.9121, 62.3267) (-383.9121, 62.2644) (-383.7961, 62.188) (-383.6235, 62.1343) knots 0 0 0 1 2 2 2
  spline S329 degree 2 poles (-383.6235, 62.1343) (-383.2896, 62.0381) (-382.9982, 61.7325) (-382.9982, 61.492) knots 0 0 0 1 2 2 2
  spline S330 degree 2 poles (-381.8835, 61.5995) (-381.8608, 61.4581) (-381.5836, 61.2996) (-381.3572, 61.2996) knots 0 0 0 1 2 2 2
  spline S331 degree 2 poles (-381.3572, 61.2996) (-381.0403, 61.2996) (-380.7574, 61.4213) knots 0 0 0 1 1 1
  line L366 (-380.7574, 61.4213) -> (-380.7574, 60.8469)
  spline S332 degree 2 poles (-380.7574, 60.8469) (-381.0856, 60.714) (-381.5581, 60.714) knots 0 0 0 1 1 1
  spline S333 degree 2 poles (-381.5581, 60.714) (-382.1268, 60.714) (-382.7606, 61.2968) (-382.7606, 61.8089) knots 0 0 0 1 2 2 2
  spline S334 degree 2 poles (-382.7606, 61.8089) (-382.7606, 62.1597) (-382.4833, 62.6945) (-381.9372, 63) (-381.6062, 63) knots 0 0 0 1 2 3 3 3
  spline S335 degree 2 poles (-381.6062, 63) (-381.2695, 63) (-380.7885, 62.7369) (-380.5395, 62.2588) (-380.5395, 61.9391) knots 0 0 0 1 2 3 3 3
  line L367 (-380.5395, 61.9391) -> (-380.5395, 61.5995)
  line L368 (-380.5395, 61.5995) -> (-381.8835, 61.5995)
  spline S336 degree 2 poles (-381.3402, 62.0749) (-381.3402, 62.4512) (-381.609, 62.4512) knots 0 0 0 1 1 1
  spline S337 degree 2 poles (-381.609, 62.4512) (-381.7222, 62.4512) (-381.875, 62.2446) (-381.8891, 62.0749) knots 0 0 0 1 2 2 2
  line L369 (-381.8891, 62.0749) -> (-381.3402, 62.0749)
  line L370 (-378.8137, 60.7677) -> (-378.8137, 61.956)
  spline S338 degree 2 poles (-378.8137, 61.956) (-378.8137, 62.1597) (-378.9353, 62.3352) (-379.0711, 62.3352) knots 0 0 0 1 2 2 2
  spline S339 degree 2 poles (-379.0711, 62.3352) (-379.1871, 62.3352) (-379.3201, 62.1513) (-379.3201, 62.0098) knots 0 0 0 1 2 2 2
  line L371 (-379.3201, 62.0098) -> (-379.3201, 60.7677)
  line L372 (-379.3201, 60.7677) -> (-380.2255, 60.7677)
  line L373 (-380.2255, 60.7677) -> (-380.2255, 62.9463)
  line L374 (-380.2255, 62.9463) -> (-379.3201, 62.9463)
  line L375 (-379.3201, 62.9463) -> (-379.3201, 62.6068)
  line L376 (-379.3201, 62.6068) -> (-379.3116, 62.6068)
  spline S340 degree 2 poles (-379.3116, 62.6068) (-379.2041, 62.7935) (-378.8363, 63) (-378.6213, 63) knots 0 0 0 1 2 2 2
  spline S341 degree 2 poles (-378.6213, 63) (-377.9083, 63) (-377.9083, 62.0975) knots 0 0 0 1 1 1
  line L377 (-377.9083, 62.0975) -> (-377.9083, 60.7677)
  line L378 (-377.9083, 60.7677) -> (-378.8137, 60.7677)
  spline S342 degree 2 poles (-375.9645, 60.796) (-376.0268, 60.7677) (-376.3069, 60.714) (-376.5049, 60.714) knots 0 0 0 1 2 2 2
  spline S343 degree 2 poles (-376.5049, 60.714) (-376.8841, 60.714) (-377.3113, 61.1299) (-377.3113, 61.5175) knots 0 0 0 1 2 2 2
  line L379 (-377.3113, 61.5175) -> (-377.3113, 62.3182)
  line L380 (-377.3113, 62.3182) -> (-377.6536, 62.3182)
  line L381 (-377.6536, 62.3182) -> (-377.6536, 62.9463)
  line L382 (-377.6536, 62.9463) -> (-377.3113, 62.9463)
  line L383 (-377.3113, 62.9463) -> (-377.3113, 63.3735)
  line L384 (-377.3113, 63.3735) -> (-376.4172, 63.6197)
  line L385 (-376.4172, 63.6197) -> (-376.4172, 62.9463)
  line L386 (-376.4172, 62.9463) -> (-375.9645, 62.9463)
  line L387 (-375.9645, 62.9463) -> (-375.9645, 62.3182)
  line L388 (-375.9645, 62.3182) -> (-376.4172, 62.3182)
  line L389 (-376.4172, 62.3182) -> (-376.4172, 61.6646)
  spline S344 degree 2 poles (-376.4172, 61.6646) (-376.4172, 61.3789) (-376.1909, 61.3789) knots 0 0 0 1 1 1
  spline S345 degree 2 poles (-376.1909, 61.3789) (-376.0834, 61.3789) (-375.9645, 61.4241) knots 0 0 0 1 1 1
  line L390 (-375.9645, 61.4241) -> (-375.9645, 60.796)
  line L391 (-375.6816, 60.7677) -> (-375.6816, 62.9463)
  line L392 (-375.6816, 62.9463) -> (-374.7762, 62.9463)
  line L393 (-374.7762, 62.9463) -> (-374.7762, 60.7677)
  line L394 (-374.7762, 60.7677) -> (-375.6816, 60.7677)
  spline S346 degree 2 poles (-374.7225, 63.5348) (-374.7225, 63.3424) (-375.0026, 63.1047) (-375.2289, 63.1047) knots 0 0 0 1 2 2 2
  spline S347 degree 2 poles (-375.2289, 63.1047) (-375.4496, 63.1047) (-375.7325, 63.3509) (-375.7325, 63.5348) knots 0 0 0 1 2 2 2
  spline S348 degree 2 poles (-375.7325, 63.5348) (-375.7325, 63.7215) (-375.4581, 63.9535) (-375.2289, 63.9535) knots 0 0 0 1 2 2 2
  spline S349 degree 2 poles (-375.2289, 63.9535) (-375.0026, 63.9535) (-374.7225, 63.7215) (-374.7225, 63.5348) knots 0 0 0 1 2 2 2
  line L395 (-372.9287, 60.7677) -> (-372.9287, 61.956)
  spline S350 degree 2 poles (-372.9287, 61.956) (-372.9287, 62.1597) (-373.0503, 62.3352) (-373.1862, 62.3352) knots 0 0 0 1 2 2 2
  spline S351 degree 2 poles (-373.1862, 62.3352) (-373.3022, 62.3352) (-373.4351, 62.1513) (-373.4351, 62.0098) knots 0 0 0 1 2 2 2
  line L396 (-373.4351, 62.0098) -> (-373.4351, 60.7677)
  line L397 (-373.4351, 60.7677) -> (-374.3405, 60.7677)
  line L398 (-374.3405, 60.7677) -> (-374.3405, 62.9463)
  line L399 (-374.3405, 62.9463) -> (-373.4351, 62.9463)
  line L400 (-373.4351, 62.9463) -> (-373.4351, 62.6068)
  line L401 (-373.4351, 62.6068) -> (-373.4266, 62.6068)
  spline S352 degree 2 poles (-373.4266, 62.6068) (-373.3191, 62.7935) (-372.9513, 63) (-372.7363, 63) knots 0 0 0 1 2 2 2
  spline S353 degree 2 poles (-372.7363, 63) (-372.0233, 63) (-372.0233, 62.0975) knots 0 0 0 1 1 1
  line L402 (-372.0233, 62.0975) -> (-372.0233, 60.7677)
  line L403 (-372.0233, 60.7677) -> (-372.9287, 60.7677)
  line L404 (-371.6131, 60.7677) -> (-371.6131, 62.9463)
  line L405 (-371.6131, 62.9463) -> (-370.7077, 62.9463)
  line L406 (-370.7077, 62.9463) -> (-370.7077, 60.7677)
  line L407 (-370.7077, 60.7677) -> (-371.6131, 60.7677)
  spline S354 degree 2 poles (-370.6539, 63.5348) (-370.6539, 63.3424) (-370.934, 63.1047) (-371.1604, 63.1047) knots 0 0 0 1 2 2 2
  spline S355 degree 2 poles (-371.1604, 63.1047) (-371.3811, 63.1047) (-371.664, 63.3509) (-371.664, 63.5348) knots 0 0 0 1 2 2 2
  spline S356 degree 2 poles (-371.664, 63.5348) (-371.664, 63.7215) (-371.3895, 63.9535) (-371.1604, 63.9535) knots 0 0 0 1 2 2 2
  spline S357 degree 2 poles (-371.1604, 63.9535) (-370.934, 63.9535) (-370.6539, 63.7215) (-370.6539, 63.5348) knots 0 0 0 1 2 2 2
  line L408 (-367.0663, 60.7677) -> (-367.1993, 61.3279)
  line L409 (-367.1993, 61.3279) -> (-368.1104, 61.3279)
  line L410 (-368.1104, 61.3279) -> (-368.2547, 60.7677)
  line L411 (-368.2547, 60.7677) -> (-369.2477, 60.7677)
  line L412 (-369.2477, 60.7677) -> (-368.1981, 63.8177)
  line L413 (-368.1981, 63.8177) -> (-367.0579, 63.8177)
  line L414 (-367.0579, 63.8177) -> (-366.0676, 60.7677)
  line L415 (-366.0676, 60.7677) -> (-367.0663, 60.7677)
  line L416 (-367.6435, 63.1528) -> (-367.6633, 63.1528)
  spline S358 degree 2 poles (-367.6633, 63.1528) (-367.669, 63.1019) (-367.7199, 62.8671) (-367.9519, 61.9815) knots 0 0 0 1 2 2 2
  line L417 (-367.9519, 61.9815) -> (-367.3691, 61.9815)
  line L418 (-367.3691, 61.9815) -> (-367.5813, 62.8105)
  spline S359 degree 2 poles (-367.5813, 62.8105) (-367.6266, 62.9944) (-367.6435, 63.1528) knots 0 0 0 1 1 1
  line L419 (-365.7932, 60.7677) -> (-365.7932, 63.9931)
  line L420 (-365.7932, 63.9931) -> (-364.8878, 63.9931)
  line L421 (-364.8878, 63.9931) -> (-364.8878, 60.7677)
  line L422 (-364.8878, 60.7677) -> (-365.7932, 60.7677)
  spline S360 degree 2 poles (-363.6712, 61.5995) (-363.6485, 61.4581) (-363.3713, 61.2996) (-363.1449, 61.2996) knots 0 0 0 1 2 2 2
  spline S361 degree 2 poles (-363.1449, 61.2996) (-362.828, 61.2996) (-362.5451, 61.4213) knots 0 0 0 1 1 1
  line L423 (-362.5451, 61.4213) -> (-362.5451, 60.8469)
  spline S362 degree 2 poles (-362.5451, 60.8469) (-362.8733, 60.714) (-363.3458, 60.714) knots 0 0 0 1 1 1
  spline S363 degree 2 poles (-363.3458, 60.714) (-363.9145, 60.714) (-364.5483, 61.2968) (-364.5483, 61.8089) knots 0 0 0 1 2 2 2
  spline S364 degree 2 poles (-364.5483, 61.8089) (-364.5483, 62.1597) (-364.271, 62.6945) (-363.7249, 63) (-363.3939, 63) knots 0 0 0 1 2 3 3 3
  spline S365 degree 2 poles (-363.3939, 63) (-363.0572, 63) (-362.5762, 62.7369) (-362.3272, 62.2588) (-362.3272, 61.9391) knots 0 0 0 1 2 3 3 3
  line L424 (-362.3272, 61.9391) -> (-362.3272, 61.5995)
  line L425 (-362.3272, 61.5995) -> (-363.6712, 61.5995)
  spline S366 degree 2 poles (-363.1279, 62.0749) (-363.1279, 62.4512) (-363.3967, 62.4512) knots 0 0 0 1 1 1
  spline S367 degree 2 poles (-363.3967, 62.4512) (-363.5099, 62.4512) (-363.6627, 62.2446) (-363.6768, 62.0749) knots 0 0 0 1 2 2 2
  line L426 (-363.6768, 62.0749) -> (-363.1279, 62.0749)
  spline S368 degree 2 poles (-360.242, 61.492) (-360.242, 61.1214) (-360.8079, 60.714) (-361.3115, 60.714) knots 0 0 0 1 2 2 2
  spline S369 degree 2 poles (-361.3115, 60.714) (-361.4586, 60.714) (-361.8915, 60.7734) (-362.0273, 60.8158) knots 0 0 0 1 2 2 2
  line L427 (-362.0273, 60.8158) -> (-362.0273, 61.4524)
  spline S370 degree 2 poles (-362.0273, 61.4524) (-361.6256, 61.2742) (-361.354, 61.2742) knots 0 0 0 1 1 1
  spline S371 degree 2 poles (-361.354, 61.2742) (-361.088, 61.2742) (-361.088, 61.4128) knots 0 0 0 1 1 1
  spline S372 degree 2 poles (-361.088, 61.4128) (-361.088, 61.4694) (-361.2125, 61.5458) (-361.4728, 61.6307) knots 0 0 0 1 2 2 2
  spline S373 degree 2 poles (-361.4728, 61.6307) (-361.7642, 61.724) (-362.0273, 62.0268) (-362.0273, 62.2673) knots 0 0 0 1 2 2 2
  spline S374 degree 2 poles (-362.0273, 62.2673) (-362.0273, 62.6068) (-361.4869, 63) (-361.0003, 63) knots 0 0 0 1 2 2 2
  spline S375 degree 2 poles (-361.0003, 63) (-360.7145, 63) (-360.3948, 62.918) knots 0 0 0 1 1 1
  line L428 (-360.3948, 62.918) -> (-360.3948, 62.3069)
  spline S376 degree 2 poles (-360.3948, 62.3069) (-360.5306, 62.3635) (-360.8503, 62.4398) (-360.9579, 62.4398) knots 0 0 0 1 2 2 2
  spline S377 degree 2 poles (-360.9579, 62.4398) (-361.0484, 62.4398) (-361.1559, 62.3804) (-361.1559, 62.3267) knots 0 0 0 1 2 2 2
  spline S378 degree 2 poles (-361.1559, 62.3267) (-361.1559, 62.2644) (-361.0399, 62.188) (-360.8673, 62.1343) knots 0 0 0 1 2 2 2
  spline S379 degree 2 poles (-360.8673, 62.1343) (-360.5335, 62.0381) (-360.242, 61.7325) (-360.242, 61.492) knots 0 0 0 1 2 2 2
  spline S380 degree 2 poles (-358.137, 61.492) (-358.137, 61.1214) (-358.7029, 60.714) (-359.2065, 60.714) knots 0 0 0 1 2 2 2
  spline S381 degree 2 poles (-359.2065, 60.714) (-359.3536, 60.714) (-359.7865, 60.7734) (-359.9223, 60.8158) knots 0 0 0 1 2 2 2
  line L429 (-359.9223, 60.8158) -> (-359.9223, 61.4524)
  spline S382 degree 2 poles (-359.9223, 61.4524) (-359.5206, 61.2742) (-359.249, 61.2742) knots 0 0 0 1 1 1
  spline S383 degree 2 poles (-359.249, 61.2742) (-358.983, 61.2742) (-358.983, 61.4128) knots 0 0 0 1 1 1
  spline S384 degree 2 poles (-358.983, 61.4128) (-358.983, 61.4694) (-359.1075, 61.5458) (-359.3678, 61.6307) knots 0 0 0 1 2 2 2
  spline S385 degree 2 poles (-359.3678, 61.6307) (-359.6592, 61.724) (-359.9223, 62.0268) (-359.9223, 62.2673) knots 0 0 0 1 2 2 2
  spline S386 degree 2 poles (-359.9223, 62.2673) (-359.9223, 62.6068) (-359.3819, 63) (-358.8953, 63) knots 0 0 0 1 2 2 2
  spline S387 degree 2 poles (-358.8953, 63) (-358.6095, 63) (-358.2898, 62.918) knots 0 0 0 1 1 1
  line L430 (-358.2898, 62.918) -> (-358.2898, 62.3069)
  spline S388 degree 2 poles (-358.2898, 62.3069) (-358.4256, 62.3635) (-358.7453, 62.4398) (-358.8529, 62.4398) knots 0 0 0 1 2 2 2
  spline S389 degree 2 poles (-358.8529, 62.4398) (-358.9434, 62.4398) (-359.0509, 62.3804) (-359.0509, 62.3267) knots 0 0 0 1 2 2 2
  spline S390 degree 2 poles (-359.0509, 62.3267) (-359.0509, 62.2644) (-358.9349, 62.188) (-358.7623, 62.1343) knots 0 0 0 1 2 2 2
  spline S391 degree 2 poles (-358.7623, 62.1343) (-358.4285, 62.0381) (-358.137, 61.7325) (-358.137, 61.492) knots 0 0 0 1 2 2 2
  line L431 (-356.5951, 60.7677) -> (-356.5951, 61.0987)
  line L432 (-356.5951, 61.0987) -> (-356.6035, 61.0987)
  spline S392 degree 2 poles (-356.6035, 61.0987) (-356.8214, 60.714) (-357.2684, 60.714) knots 0 0 0 1 1 1
  spline S393 degree 2 poles (-357.2684, 60.714) (-357.5768, 60.714) (-357.9248, 61.0789) (-357.9248, 61.3873) knots 0 0 0 1 2 2 2
  spline S394 degree 2 poles (-357.9248, 61.3873) (-357.9248, 62.0296) (-357.1355, 62.1314) knots 0 0 0 1 1 1
  line L433 (-357.1355, 62.1314) -> (-356.5951, 62.2022)
  spline S395 degree 2 poles (-356.5951, 62.2022) (-356.5951, 62.3097) (-356.7875, 62.4455) (-356.9487, 62.4455) knots 0 0 0 1 2 2 2
  spline S396 degree 2 poles (-356.9487, 62.4455) (-357.3137, 62.4455) (-357.7211, 62.2361) knots 0 0 0 1 1 1
  line L434 (-357.7211, 62.2361) -> (-357.7211, 62.8246)
  spline S397 degree 2 poles (-357.7211, 62.8246) (-357.5457, 62.901) (-357.011, 63) (-356.8214, 63) knots 0 0 0 1 2 2 2
  spline S398 degree 2 poles (-356.8214, 63) (-356.2669, 63) (-355.7661, 62.5247) (-355.7661, 61.9702) knots 0 0 0 1 2 2 2
  line L435 (-355.7661, 61.9702) -> (-355.7661, 60.7677)
  line L436 (-355.7661, 60.7677) -> (-356.5951, 60.7677)
  spline S399 degree 2 poles (-357.1326, 61.509) (-357.1326, 61.4213) (-357.0195, 61.3053) (-356.9148, 61.3053) knots 0 0 0 1 2 2 2
  spline S400 degree 2 poles (-356.9148, 61.3053) (-356.7733, 61.3053) (-356.5951, 61.5175) (-356.5951, 61.6844) knots 0 0 0 1 2 2 2
  line L437 (-356.5951, 61.6844) -> (-356.5951, 61.7665)
  line L438 (-356.5951, 61.7665) -> (-356.9035, 61.724)
  spline S401 degree 2 poles (-356.9035, 61.724) (-357.1326, 61.6844) (-357.1326, 61.509) knots 0 0 0 1 1 1
  line L439 (-353.9468, 60.7677) -> (-353.9468, 61.956)
  spline S402 degree 2 poles (-353.9468, 61.956) (-353.9468, 62.1597) (-354.0685, 62.3352) (-354.2043, 62.3352) knots 0 0 0 1 2 2 2
  spline S403 degree 2 poles (-354.2043, 62.3352) (-354.3203, 62.3352) (-354.4533, 62.1513) (-354.4533, 62.0098) knots 0 0 0 1 2 2 2
  line L440 (-354.4533, 62.0098) -> (-354.4533, 60.7677)
  line L441 (-354.4533, 60.7677) -> (-355.3586, 60.7677)
  line L442 (-355.3586, 60.7677) -> (-355.3586, 62.9463)
  line L443 (-355.3586, 62.9463) -> (-354.4533, 62.9463)
  line L444 (-354.4533, 62.9463) -> (-354.4533, 62.6068)
  line L445 (-354.4533, 62.6068) -> (-354.4448, 62.6068)
  spline S404 degree 2 poles (-354.4448, 62.6068) (-354.3373, 62.7935) (-353.9695, 63) (-353.7544, 63) knots 0 0 0 1 2 2 2
  spline S405 degree 2 poles (-353.7544, 63) (-353.0414, 63) (-353.0414, 62.0975) knots 0 0 0 1 1 1
  line L446 (-353.0414, 62.0975) -> (-353.0414, 60.7677)
  line L447 (-353.0414, 60.7677) -> (-353.9468, 60.7677)
  line L448 (-351.1769, 60.7677) -> (-351.1769, 61.0224)
  line L449 (-351.1769, 61.0224) -> (-351.1854, 61.0224)
  spline S406 degree 2 poles (-351.1854, 61.0224) (-351.2929, 60.8781) (-351.6438, 60.714) (-351.8135, 60.714) knots 0 0 0 1 2 2 2
  spline S407 degree 2 poles (-351.8135, 60.714) (-352.0908, 60.714) (-352.518, 60.9884) (-352.7274, 61.4835) (-352.7274, 61.8174) knots 0 0 0 1 2 3 3 3
  spline S408 degree 2 poles (-352.7274, 61.8174) (-352.7274, 62.1654) (-352.4756, 62.703) (-352.0201, 63) (-351.7371, 63) knots 0 0 0 1 2 3 3 3
  spline S409 degree 2 poles (-351.7371, 63) (-351.6041, 63) (-351.3778, 62.9237) (-351.208, 62.7935) (-351.1854, 62.7284) knots 0 0 0 1 2 3 3 3
  line L450 (-351.1854, 62.7284) -> (-351.1769, 62.7284)
  line L451 (-351.1769, 62.7284) -> (-351.1769, 63.9931)
  line L452 (-351.1769, 63.9931) -> (-350.2715, 63.9931)
  line L453 (-350.2715, 63.9931) -> (-350.2715, 60.7677)
  line L454 (-350.2715, 60.7677) -> (-351.1769, 60.7677)
  spline S410 degree 2 poles (-351.1571, 61.9221) (-351.1571, 62.1173) (-351.3297, 62.3352) (-351.4768, 62.3352) knots 0 0 0 1 2 2 2
  spline S411 degree 2 poles (-351.4768, 62.3352) (-351.624, 62.3352) (-351.8079, 62.0664) (-351.8079, 61.84) knots 0 0 0 1 2 2 2
  spline S412 degree 2 poles (-351.8079, 61.84) (-351.8079, 61.3789) (-351.4881, 61.3789) knots 0 0 0 1 1 1
  spline S413 degree 2 poles (-351.4881, 61.3789) (-351.3382, 61.3789) (-351.1571, 61.6278) (-351.1571, 61.8655) knots 0 0 0 1 2 2 2
  line L455 (-351.1571, 61.8655) -> (-351.1571, 61.9221)
  spline S414 degree 2 poles (-348.1948, 62.1711) (-348.2458, 62.1937) (-348.4212, 62.2305) (-348.4778, 62.2305) knots 0 0 0 1 2 2 2
  spline S415 degree 2 poles (-348.4778, 62.2305) (-348.9276, 62.2305) (-348.9276, 61.7127) knots 0 0 0 1 1 1
  line L456 (-348.9276, 61.7127) -> (-348.9276, 60.7677)
  line L457 (-348.9276, 60.7677) -> (-349.833, 60.7677)
  line L458 (-349.833, 60.7677) -> (-349.833, 62.9463)
  line L459 (-349.833, 62.9463) -> (-348.9276, 62.9463)
  line L460 (-348.9276, 62.9463) -> (-348.9276, 62.5643)
  line L461 (-348.9276, 62.5643) -> (-348.9191, 62.5643)
  spline S416 degree 2 poles (-348.9191, 62.5643) (-348.8371, 62.7709) (-348.5287, 62.9859) (-348.325, 62.9859) knots 0 0 0 1 2 2 2
  spline S417 degree 2 poles (-348.325, 62.9859) (-348.2514, 62.9859) (-348.1948, 62.9604) knots 0 0 0 1 1 1
  line L462 (-348.1948, 62.9604) -> (-348.1948, 62.1711)
  spline S418 degree 2 poles (-345.5126, 61.8966) (-345.5126, 61.3449) (-346.1775, 60.714) (-346.7745, 60.714) knots 0 0 0 1 2 2 2